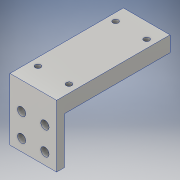
# Autodesk Inventor part: SupportForStopAirCylinder
Saved by Autodesk Inventor 2016 (Build 200138000, 138)
## iProperties
Created: 2015-07-18
Part Number: SupportForStopAirCylinder
Material: Aluminum 6061
Document SubType Name: Modeling
Designer: steele
Density: 2.7 g/cm^3
Appearance: Aluminum - Flat
Mass: 141.373 g
Surface Area: 146.17 cm^2
Volume: 52.3602 cm^3
Author: steele
Autodesk Inventor part; units mm, degrees
ref_plane "YZ Plane" through (0, 0, 0) normal (1, 0, 0) x (0, 1, 0)
ref_plane "XZ Plane" through (0, 0, 0) normal (0, 1, 0) x (-1, 0, 0)
ref_plane "XY Plane" through (0, 0, 0) normal (0, 0, 1) x (1, 0, 0)
sketch "Sketch2" plane through (0, 0, 0) normal (0, 1, 0) x (-1, 0, 0)
  line L0 (-19.05, 44.45) -> (-19.05, -44.45)
  line L1 (-19.05, -44.45) -> (19.05, -44.45)
  line L2 (19.05, -44.45) -> (19.05, 44.45)
  line L3 (19.05, 44.45) -> (-19.05, 44.45) construction
  line L4 (-19.05, 44.45) -> (19.05, -44.45) construction
  line L5 (-19.05, -44.45) -> (19.05, 44.45) construction
  line L6 (19.05, 44.45) -> (19.05, 48.26)
  line L7 (19.05, 48.26) -> (-19.05, 48.26)
  line L8 (-19.05, 48.26) -> (-19.05, 43.3404)
  point P0 (0, 0)
  dimension "lengthBaseAirCylinder" = 88.9
  dimension "widthBaseOfAirCylinder" = 38.1
  dimension "extenstionForStroke" = 3.81
  constraints: 18 end point, 3 parallel, 2 midpoint, 2 perpendicular, 2 vertical, 1 point on line
  measures "lengthBaseAirCylinder" distance of L0.start L0.end
  measures "widthBaseOfAirCylinder" distance of L0.end L1.end
  measures "extenstionForStroke" distance between parallel lines of L7 L3
extrude "Extrusion1" add sketch "Sketch2" against normal blind 12.7
sketch "Sketch3" plane through (0, -12.7, 0) normal (0, -1, 0) x (1, 0, 0)
  line L0 (19.05, -44.45) -> (19.05, 48.26) projected
  line L1 (-19.05, 48.26) -> (-19.05, -44.45) projected
  line L2 (19.05, 48.26) -> (-19.05, 48.26)
  line L3 (-19.05, 48.26) -> (-19.05, 41.91)
  line L4 (-19.05, 41.91) -> (19.05, 41.91)
  line L5 (19.05, 41.91) -> (19.05, 48.26)
  point P0 (0, 0)
  dimension "d9" = 6.35
  constraints: 8 end point, 2 parallel, 1 horizontal, 1 perpendicular, 1 point on line
  measures "d9" distance between parallel lines of L4 L2
extrude "Extrusion2" add sketch "Sketch3" along normal blind 38.1
sketch "Sketch4" plane through (0, 0, 0) normal (0, 1, 0) x (1, 0, 0)
  line L0 (12.7, -31.75) -> (12.7, 31.75) construction
  line L1 (12.7, 31.75) -> (-12.7, 31.75) construction
  line L2 (-12.7, 31.75) -> (-12.7, -31.75) construction
  line L3 (-12.7, -31.75) -> (12.7, -31.75) construction
  line L4 (12.7, -31.75) -> (-12.7, 31.75) construction
  line L5 (12.7, 31.75) -> (-12.7, -31.75) construction
  point P0 (0, 0)
  dimension "widthForCylinderBoltHoles" = 25.4
  dimension "lengthForCylinderHoles" = 63.5
  constraints: 12 end point, 4 coincident, 2 midpoint, 2 parallel, 1 perpendicular, 1 vertical
  measures "widthForCylinderBoltHoles" distance of L0.end L1.end
  measures "lengthForCylinderHoles" distance of L1.end L2.end
hole "Hole1" at (12.7, 0, 31.75) at (12.7, 0, -31.75) at (-12.7, 0, -31.75) at (-12.7, 0, 31.75) direction (0, -1, 0) diameter 4.4958 end through all clearance for "Flat Head Machine Screw (82)" size "#8" standard "Ansi Unified Screw Threads"
sketch "Sketch5" plane through (-19.05, 0, 48.26) normal (0, 0, 1) x (1, 0, 0)
  line L0 (38.1, -12.7) -> (0, -12.7) projected
  line L1 (19.05, -12.7) -> (19.05, -50.8) construction
  line L2 (38.1, -50.8) -> (0, -50.8) construction
  line L3 (9.525, -41.275) -> (28.575, -41.275) construction
  line L4 (28.575, -41.275) -> (28.575, -22.225) construction
  line L5 (28.575, -22.225) -> (9.525, -22.225) construction
  line L6 (9.525, -22.225) -> (9.525, -41.275) construction
  line L7 (9.525, -41.275) -> (28.575, -22.225) construction
  line L8 (28.575, -41.275) -> (9.525, -22.225) construction
  point P0 (19.05, 0)
  point P1 (19.05, -31.75)
  dimension "d21" = 19.05
  dimension "d22" = 19.05
  constraints: 14 end point, 5 midpoint, 4 coincident, 2 parallel, 1 horizontal, 1 perpendicular
  measures "d21" distance of L3.start L3.end
  measures "d22" distance of L3.end L4.end
hole "Hole2" at (-9.525, -41.275, 48.26) at (9.525, -41.275, 48.26) at (9.525, -22.225, 48.26) at (-9.525, -22.225, 48.26) direction (0, 0, -1) diameter 6.7564 end through all clearance for "Flat Head Machine Screw (82)" size "1/4" standard "Ansi Unified Screw Threads"
body "Solid1"
